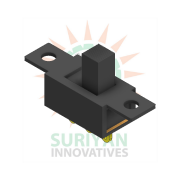
# Autodesk Inventor part: Sliding Switch own made
Saved by Autodesk Inventor 2020 (Build 240168000, 168)
## iProperties
Created: 2019-10-08
Part Number: Sliding Switch own made
Material: Generic
Document SubType Name: Modeling
Designer: Suriyan.S
Density: 1 g/cm^3
Appearance: Default
Author: Suriyan.S
Autodesk Inventor part; units mm, degrees
ref_plane "YZ Plane" through (0, 0, 0) normal (1, 0, 0) x (0, 1, 0)
ref_plane "XZ Plane" through (0, 0, 0) normal (0, 1, 0) x (-1, 0, 0)
ref_plane "XY Plane" through (0, 0, 0) normal (0, 0, 1) x (1, 0, 0)
sketch "Sketch1" plane through (0, 0, 0) normal (0, 0, 1) x (1, 0, 0)
  line L0 (-5.25, -2.5) -> (5.25, -2.5)
  line L1 (5.25, -2.5) -> (5.25, 2.5)
  line L2 (5.25, 2.5) -> (-5.25, 2.5)
  line L3 (-5.25, 2.5) -> (-5.25, -2.5)
  line L4 (-5.25, -2.5) -> (5.25, 2.5) construction
  line L5 (5.25, -2.5) -> (-5.25, 2.5) construction
  point P0 (0, 0)
  dimension "d0" = 5
  dimension "d1" = 10.5
  constraints: 12 end point, 2 midpoint, 2 parallel, 1 horizontal, 1 perpendicular
  measures "d0" distance of L2.end L0.start
  measures "d1" distance of L0.start L0.end
extrude "Extrusion1" add sketch "Sketch1" along normal mid plane 6
sketch "Sketch3" plane through (0, 0, 0) normal (0, 1, 0) x (-1, 0, 0)
  point P0 (0, 0)
sketch "Sketch4" plane through (-5.25, 2.5, 3) normal (0, 1, 0) x (1, 0, 0)
  line L0 (0, 6) -> (0, 0) projected
  line L1 (10.5, 6) -> (10.5, 0) projected
  line L2 (10.5, 6) -> (10.5, 0) projected
  line L3 (10.5, 5.25) -> (15, 5.25)
  line L4 (15, 5.25) -> (15, 0.75)
  line L5 (15, 0.75) -> (10.5, 0.75)
  line L6 (10.5, 0.75) -> (10.5, 5.25)
  line L7 (0, 5.25) -> (-4.5, 5.25)
  line L8 (-4.5, 5.25) -> (-4.5, 0.75)
  line L9 (-4.5, 0.75) -> (0, 0.75)
  line L10 (0, 0.75) -> (0, 5.25)
  point P0 (5.25, 3)
  point P1 (-4.5, 3)
  dimension "d4" = 4.5
  dimension "d5" = 4.5
  constraints: 16 end point, 4 parallel, 4 point on line, 2 horizontal, 2 perpendicular, 1 collinear, 1 horizontal alignment, 1 midpoint
  measures "d4" distance of L7.end L8.end
  measures "d5" distance of L7.start L7.end
extrude "Extrusion2" add sketch "Sketch4" against normal blind 0.5
sketch "Sketch5" plane through (-5.25, 2.5, 3) normal (0, 1, 0) x (1, 0, 0)
  circle A0 centre (-2.25, 3) radius 1
  circle A1 centre (12.75, 3) radius 1
  point P0 (5.25, 3)
  dimension "d8" = 2
  dimension "d9" = 2
  constraints: 2 centre point
  measures "d8" diameter of A0
  measures "d9" diameter of A1
extrude "Extrusion3" cut sketch "Sketch5" against normal blind 0.5
sketch "Sketch6" plane through (-5.25, 2.5, 3) normal (0, 1, 0) x (1, 0, 0)
  line L0 (2.25, 1.25) -> (8.25, 1.25)
  line L1 (8.25, 1.25) -> (8.25, 4.75)
  line L2 (8.25, 4.75) -> (2.25, 4.75)
  line L3 (2.25, 4.75) -> (2.25, 1.25)
  line L4 (2.25, 1.25) -> (8.25, 4.75) construction
  line L5 (8.25, 1.25) -> (2.25, 4.75) construction
  point P0 (5.25, 3)
  dimension "d12" = 3.5
  dimension "d13" = 6
  constraints: 12 end point, 2 midpoint, 2 parallel, 1 horizontal, 1 perpendicular
  measures "d12" distance of L0.end L1.end
  measures "d13" distance of L0.start L0.end
extrude "Extrusion4" cut sketch "Sketch6" against normal blind 0.5
sketch "Sketch7" plane through (-5.25, 2, 3) normal (0, 1, 0) x (1, 0, 0)
  line L0 (2.25, 4.75) -> (8.25, 4.75) projected
  line L1 (8.25, 1.25) -> (2.25, 1.25) projected
  line L2 (8.25, 4.75) -> (8.25, 1.25) projected
  line L3 (8.25, 4.5) -> (5.25, 4.5)
  line L4 (5.25, 4.5) -> (5.25, 1.5)
  line L5 (5.25, 1.5) -> (8.25, 1.5)
  line L6 (8.25, 1.5) -> (8.25, 4.5)
  point P0 (5.25, 3)
  point P1 (8.25, 1.5)
  point P2 (5.25, 4.5)
  dimension "d16" = 0.25
  dimension "d17" = 3
  dimension "d18" = 3
  constraints: 8 end point, 2 parallel, 1 horizontal, 1 perpendicular, 1 point on line
  measures "d16" distance between parallel lines of L1 L5
  measures "d17" distance of L3.end L4.end
  measures "d18" distance of L3.start L3.end
extrude "Extrusion5" add sketch "Sketch7" along normal blind 5.5
sketch "Sketch8" plane through (0, 0, 0) normal (0, 0, 1) x (1, 0, 0)
  line L0 (0, 0) -> (0, -4.75) construction
  line L1 (-0.75, 0) -> (-0.75, -4.75)
  line L2 (0.75, -4.75) -> (0.75, 0)
  arc A0 (0.75, 0) -> (-0.75, 0) centre (0, 0) ccw
  arc A1 (-0.75, -4.75) -> (0.75, -4.75) centre (0, -4.75) ccw
  line L3 (-5.25, -2.5) -> (5.25, -2.5) projected
  line L4 (0, -4.75) -> (0, -3.5146) construction
  line L5 (-0.3, -4.75) -> (-0.3, -3.5146)
  line L6 (0.3, -3.5146) -> (0.3, -4.75)
  arc A2 (-0.3, -4.75) -> (0.3, -4.75) centre (0, -4.75) ccw
  arc A3 (0.3, -3.5146) -> (-0.3, -3.5146) centre (0, -3.5146) ccw
  point P0 (0, -2.375)
  point P1 (0, -4.1323)
  point P2 (0.75, -2.5)
  point P3 (-0.75, -2.5)
  dimension "d21" = 2.25
  dimension "d22" = 0.75
  dimension "d23" = 0.3
  constraints: 16 end point, 8 point on circle, 8 tangent, 4 centre point, 2 midpoint, 2 parallel, 1 point on line, 1 vertical
  measures "d21" distance from line of L3 L0.end
  measures "d22" radius of A1
  measures "d23" radius of A2
extrude "Extrusion6" add sketch "Sketch8" along normal mid plane 0.5 contours L3 L2 A1 L1
pattern_linear "Rectangular Pattern1" count 2 spacing 3 along (1, 0, 0) count 2 spacing 3 along (-1, 0, 0) of "Extrusion6"
sketch "Sketch9" plane through (0, 2, 1.5) normal (0, 0, 1) x (1, 0, 0)
  line L0 (3, 5.5) -> (0, 5.5) projected
  circle A0 centre (1.5, 5.5) radius 0.1
  point P0 (0, -2)
  dimension "d32" = 0.2
  constraints: 1 centre point, 1 midpoint
  measures "d32" diameter of A0
extrude "Extrusion7" add sketch "Sketch9" against normal blind 3
pattern_linear "Rectangular Pattern2" count 8 spacing 0.2 along (1, 0, 0) count 8 spacing 0.2 along (-1, 0, 0) of "Extrusion7"
fillet "Fillet1" radius 0.2 4 edges at (9.75, 2.25, 2.25) (9.75, 2.25, -2.25) (-9.75, 2.25, 2.25) (-9.75, 2.25, -2.25)
sketch "Sketch10" plane through (-5.25, -2.5, -3) normal (-1, 0, 0) x (0, 0, 1)
  line L0 (5.25, 4.6131) -> (1.4151, 4.6131)
  line L1 (0.75, 4.1131) -> (5.25, 4.1131)
  line L2 (5.25, 4.5) -> (5.25, 0.5)
  line L3 (5.25, 0.5) -> (0.75, 0.5)
  line L4 (0.75, 0.5) -> (0.75, 4.1131)
  line L5 (0, 0) -> (0, 5) projected
  line L6 (6, 0) -> (0, 0) projected
  line L7 (6, 5) -> (6, 0) projected
  point P0 (3, 2.5)
  point P1 (5.25, 4.5)
  dimension "d44" = 0.75
  dimension "d45" = 0.75
  dimension "d46" = 0.5
  dimension "d47" = 0.5
  constraints: 10 end point, 2 parallel, 1 horizontal, 1 perpendicular, 1 point on line
  measures "d44" distance between parallel lines of L4 L5
  measures "d45" distance between parallel lines of L7 L2
  measures "d46" distance between parallel lines of L1 L0
  measures "d47" distance between parallel lines of L6 L3
extrude "Extrusion8" cut sketch "Sketch10" against normal blind 3
sketch "Sketch11" plane through (5.25, -2.5, 3) normal (1, 0, 0) x (0, 0, -1)
  line L0 (5.25, 4.1131) -> (0.75, 4.1131) projected
  line L1 (5.25, 0.5) -> (5.25, 4.1131) projected
  line L2 (0.75, 0.5) -> (5.25, 0.5) projected
  line L3 (0.75, 4.1131) -> (0.75, 0.5) projected
  point P0 (3, 2.5)
extrude "Extrusion9" cut sketch "Sketch11" against normal blind 0.5
body "Solid1"
